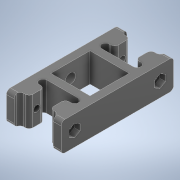
# Autodesk Inventor part: pullitens
Saved by Autodesk Inventor 2022 (Build 260153000, 153)
## iProperties
Created: 2022-03-11
Part Number: pullitens
Material: Genérico
Document SubType Name: Modeling
Designer: JK
Density: 1 g/cm^3
Appearance: Suave - Negro
Author: JK
Autodesk Inventor part; units mm, degrees
ref_plane "YZ Plane" through (0, 0, 0) normal (1, 0, 0) x (0, 1, 0)
ref_plane "XZ Plane" through (0, 0, 0) normal (0, 1, 0) x (-1, 0, 0)
ref_plane "XY Plane" through (0, 0, 0) normal (0, 0, 1) x (1, 0, 0)
sketch "Boceto1" plane through (0, 0, 0) normal (0, 1, 0) x (-1, 0, 0)
  line L0 (-10.15, 10.15) -> (10.15, 10.15)
  line L1 (10.15, 10.15) -> (10.15, -10.15)
  line L2 (10.15, -10.15) -> (-10.15, -10.15)
  line L3 (-10.15, -10.15) -> (-10.15, 10.15)
  line L4 (-10.15, 10.15) -> (10.15, -10.15) construction
  line L5 (10.15, 10.15) -> (-10.15, -10.15) construction
  line L6 (-14.15, 14.15) -> (14.15, 14.15)
  line L7 (14.15, 14.15) -> (14.15, -14.15)
  line L8 (14.15, -14.15) -> (-14.15, -14.15)
  line L9 (-14.15, -14.15) -> (-14.15, 14.15)
  line L10 (-14.15, 14.15) -> (14.15, -14.15) construction
  line L11 (14.15, 14.15) -> (-14.15, -14.15) construction
  point P0 (0, 0)
  dimension "d0" = 20.3
  dimension "d1" = 4
  constraints: 24 end point, 4 midpoint, 4 parallel, 3 perpendicular, 2 horizontal, 1 point on line
  measures "d0" distance of L0.start L0.end
  measures "d1" distance between parallel lines of L0 L6
extrude "Extrusión1" add sketch "Boceto1" along normal blind 15
sketch "Boceto3" plane through (0, 15, 0) normal (0, 1, 0) x (1, 0, 0)
  line L0 (-14.15, -29.15) -> (-10.15, -29.15)
  line L1 (-10.15, -29.15) -> (-10.15, 29.15)
  line L2 (-10.15, 29.15) -> (-14.15, 29.15)
  line L3 (-14.15, 29.15) -> (-14.15, -29.15)
  line L4 (14.15, 29.15) -> (10.15, 29.15)
  line L5 (10.15, 29.15) -> (10.15, -29.15)
  line L6 (10.15, -29.15) -> (14.15, -29.15)
  line L7 (14.15, -29.15) -> (14.15, 29.15)
  line L8 (14.15, 14.15) -> (-14.15, 14.15) projected
  line L9 (-14.15, 14.15) -> (-14.15, -14.15) projected
  line L10 (-14.15, -14.15) -> (14.15, -14.15) projected
  line L11 (14.15, -14.15) -> (14.15, 14.15) projected
  line L12 (10.15, -10.15) -> (-10.15, -10.15) projected
  line L13 (-10.15, -10.15) -> (-10.15, 10.15) projected
  line L14 (-10.15, 10.15) -> (10.15, 10.15) projected
  line L15 (10.15, 10.15) -> (10.15, -10.15) projected
  line L16 (10.15, 10.15) -> (10.15, -10.15) projected
  point P0 (-10.15, 14.15)
  point P1 (-10.15, -14.15)
  point P2 (10.15, 14.15)
  point P3 (10.15, -14.15)
  dimension "d11" = 15
  dimension "d12" = 15
  constraints: 16 end point, 5 collinear, 4 parallel, 2 horizontal, 2 perpendicular, 1 point on line
  measures "d11" distance between parallel lines of L10 L0
  measures "d12" distance between parallel lines of L2 L8
extrude "Extrusión2" add sketch "Boceto3" against normal up to surface (15 mm away) contours L3 L10 L1 L0 | L3 L2 L1 L8 | L10 L7 L6 L5 | L5 L4 L7 L8
sketch "Boceto4" plane through (-14.15, 15, -29.15) normal (-1, 0, 0) x (0, 0, 1)
  circle A0 centre (51.3, -7.5) radius 1.65
  circle A1 centre (7, -7.5) radius 1.65
  line L0 (15, -15) -> (15, 0) projected
  line L1 (0, 0) -> (58.3, 0) projected
  point P0 (29.15, -15)
  point P1 (43.3, 0)
  dimension "d15" = 3.3
  dimension "d16" = 3.3
  dimension "d23" = 8
  dimension "d24" = 8
  dimension "d25" = 7.5
  constraints: 2 centre point, 1 horizontal alignment
  measures "d15" diameter of A1
  measures "d16" diameter of A0
  measures "d23" horizontal distance of A0.centre point (43.3, 0)
  measures "d24" horizontal distance of L0.end A1.centre
  measures "d25" distance from line of A0.centre L1
extrude "Extrusión3" cut sketch "Boceto4" against normal through all
sketch "Boceto5" plane through (-14.15, 15, -29.15) normal (-1, 0, 0) x (0, 0, 1)
  circle A0 centre (51.3, -7.5) radius 1.65 projected
  circle A1 centre (51.3, -7.5) radius 6.5
  point P0 (29.15, -15)
  dimension "d22" = 13
  constraints: 1 centre point, 1 coincident
  measures "d22" diameter of A1
sketch "Boceto6" plane through (-14.15, 15, -29.15) normal (-1, 0, 0) x (0, 0, 1)
  circle A0 centre (29.15, -7.5) radius 2.7
  line L0 (58.3, -15) -> (0, -15) projected
  point P0 (29.15, -15)
  point P1 (29.15, -15)
  dimension "d26" = 5.4
  dimension "d27" = 7.5
  constraints: 1 centre point, 1 midpoint, 1 vertical alignment
  measures "d26" diameter of A0
  measures "d27" distance from line of L0 A0.centre
extrude "Extrusión4" cut sketch "Boceto6" against normal blind 16.8
fillet "Empalme1" radius 2 8 edges at (-12.15, 15, 29.15) (12.15, 15, 29.15) (12.15, 15, -29.15) (-12.15, 15, -29.15) (12.15, 0, 29.15) (-12.15, 0, 29.15) (12.15, 0, -29.15) (-12.15, 0, -29.15)
sketch "Boceto7" plane through (14.15, 15, 27.15) normal (1, 0, 0) x (0, 0, -1)
  circle A0 centre (5, -7.5) radius 1.65 projected
  circle A1 centre (5, -7.5) radius 2.85
  circle A2 centre (49.3, -7.5) radius 1.65 projected
  circle A3 centre (49.3, -7.5) radius 2.85
  line L0 (5, -4.2091) -> (7.85, -5.8546)
  line L1 (7.85, -5.8546) -> (7.85, -9.1454)
  line L2 (7.85, -9.1454) -> (5, -10.7909)
  line L3 (5, -10.7909) -> (2.15, -9.1454)
  line L4 (2.15, -9.1454) -> (2.15, -5.8546)
  line L5 (2.15, -5.8546) -> (5, -4.2091)
  line L6 (49.3, -4.2091) -> (52.15, -5.8546)
  line L7 (52.15, -5.8546) -> (52.15, -9.1454)
  line L8 (52.15, -9.1454) -> (49.3, -10.7909)
  line L9 (49.3, -10.7909) -> (46.45, -9.1454)
  line L10 (46.45, -9.1454) -> (46.45, -5.8546)
  line L11 (46.45, -5.8546) -> (49.3, -4.2091)
  point P0 (27.15, -15)
  dimension "d31" = 5.7
  constraints: 24 end point, 4 coincident, 2 centre point, 2 tangent, 2 vertical, 1 equal radius, 26 other
  measures "d31" diameter of A1
extrude "Extrusión5" cut sketch "Boceto7" against normal blind 3 contours A0 | A1 | L1 L2 A1 | A1 L0 L1 | A1 L5 L0 | L2 L3 A1 | A1 L4 L5 | L3 L4 A1 | A2 | A3 | L7 L8 A3 | A3 L6 L7 | A3 L11 L6 | L8 L9 A3 | A3 L10 L11 | L9 L10 A3
sketch "Boceto9" plane through (0, 0, 0) normal (0, -1, 0) x (1, 0, 0)
  line L0 (-14.15, 27.15) -> (-14.15, -27.15) projected
  line L1 (-10.15, 26.15) -> (-14.15, 26.15)
  line L2 (-14.15, 26.15) -> (-14.15, 18.15)
  line L3 (-14.15, 18.15) -> (-10.15, 18.15)
  line L4 (-10.15, 18.15) -> (-10.15, 26.15)
  line L5 (-10.15, 26.15) -> (-14.15, 18.15) construction
  line L6 (-14.15, 26.15) -> (-10.15, 18.15) construction
  line L7 (-10.15, 14.15) -> (-10.15, 27.15) projected
  line L8 (-10.15, -18.15) -> (-14.15, -18.15)
  line L9 (-14.15, -18.15) -> (-14.15, -26.15)
  line L10 (-14.15, -26.15) -> (-10.15, -26.15)
  line L11 (-10.15, -26.15) -> (-10.15, -18.15)
  line L12 (-10.15, -18.15) -> (-14.15, -26.15) construction
  line L13 (-14.15, -18.15) -> (-10.15, -26.15) construction
  line L14 (-10.15, -27.15) -> (-10.15, -14.15) projected
  line L15 (14.15, 27.15) -> (14.15, -27.15) projected
  line L16 (-14.15, 26.15) -> (14.15, 26.15)
  line L17 (14.15, 26.15) -> (14.15, 18.15)
  line L18 (14.15, 18.15) -> (-14.15, 18.15)
  line L19 (-14.15, 18.15) -> (-14.15, 26.15)
  line L20 (-14.15, -18.15) -> (14.15, -18.15)
  line L21 (14.15, -18.15) -> (14.15, -26.15)
  line L22 (14.15, -26.15) -> (-14.15, -26.15)
  line L23 (-14.15, -26.15) -> (-14.15, -18.15)
  line L24 (-5.4, 26.15) -> (5.4, 26.15)
  line L25 (5.4, 26.15) -> (5.4, 18.15)
  line L26 (5.4, 18.15) -> (-5.4, 18.15)
  line L27 (-5.4, 18.15) -> (-5.4, 26.15)
  line L28 (-5.4, 26.15) -> (5.4, 18.15) construction
  line L29 (5.4, 26.15) -> (-5.4, 18.15) construction
  line L30 (-5.4, -18.15) -> (5.4, -18.15)
  line L31 (5.4, -18.15) -> (5.4, -26.15)
  line L32 (5.4, -26.15) -> (-5.4, -26.15)
  line L33 (-5.4, -26.15) -> (-5.4, -18.15)
  line L34 (-5.4, -18.15) -> (5.4, -26.15) construction
  line L35 (5.4, -18.15) -> (-5.4, -26.15) construction
  line L36 (-10.15, -27.15) -> (-14.15, -27.15) projected
  line L37 (-10.15, -27.15) -> (-10.15, -14.15) projected
  line L38 (10.15, -14.15) -> (-10.15, -14.15) projected
  line L39 (10.15, -14.15) -> (10.15, -27.15) projected
  line L40 (14.15, -27.15) -> (10.15, -27.15) projected
  line L41 (14.15, -27.15) -> (14.15, 27.15) projected
  line L42 (10.15, 27.15) -> (14.15, 27.15) projected
  line L43 (10.15, 27.15) -> (10.15, 14.15) projected
  line L44 (-10.15, 14.15) -> (10.15, 14.15) projected
  line L45 (-10.15, 14.15) -> (-10.15, 27.15) projected
  line L46 (-14.15, 27.15) -> (-10.15, 27.15) projected
  line L47 (-14.15, 27.15) -> (-14.15, -27.15) projected
  line L48 (10.15, 10.15) -> (-10.15, 10.15) projected
  line L49 (10.15, -10.15) -> (10.15, 10.15) projected
  line L50 (-10.15, -10.15) -> (10.15, -10.15) projected
  line L51 (-10.15, 10.15) -> (-10.15, -10.15) projected
  point P0 (0, 0)
  point P1 (-12.15, 22.15)
  point P2 (-12.15, -22.15)
  point P3 (0, 22.15)
  point P4 (0, -22.15)
  point P5 (0, -22.15)
  point P6 (0, 22.15)
  point P7 (10.15, -26.15)
  point P8 (10.15, -18.15)
  point P9 (-5.4, 18.15)
  point P10 (10.15, 18.15)
  point P11 (10.15, 26.15)
  dimension "d37" = 22.15
  dimension "d38" = 8
  dimension "d39" = 22.15
  dimension "d40" = 8
  dimension "d41" = 10.8
  dimension "d42" = 8
  constraints: 64 end point, 12 parallel, 10 midpoint, 7 collinear, 6 horizontal, 6 perpendicular, 5 point on line, 2 vertical alignment
  measures "d37" vertical distance of point (0, 0) point (-12.15, 22.15)
  measures "d38" distance between parallel lines of L3 L1
  measures "d39" vertical distance of point (0, 0) point (-12.15, -22.15)
  measures "d40" distance between parallel lines of L10 L8
  measures "d41" distance between parallel lines of L27 L25
  measures "d42" distance of L30.end L31.end
extrude "Extrusión7" add sketch "Boceto9" against normal up to surface (15 mm away) contours L16 L27 L18 L4 | L20 L33 L22 L11 | L16 L43 L18 L25 | L20 L39 L22 L31
sketch "Boceto10" plane through (14.15, 15, 27.15) normal (1, 0, 0) x (0, 0, -1)
  circle A0 centre (5, -7.5) radius 1.65 projected
  circle A1 centre (49.3, -7.5) radius 1.65 projected
  point P0 (27.15, -15)
extrude "Extrusión8" cut sketch "Boceto10" against normal through all
fillet "Empalme2" radius 2 20 edges at (10.15, 7.5, 18.15) (10.15, 7.5, 26.15) (10.15, 7.5, -18.15) (10.15, 7.5, -26.15) (10.15, 7.5, -14.15) (-10.15, 7.5, -14.15) (-10.15, 7.5, -18.15) (-10.15, 7.5, -26.15) (-10.15, 7.5, 18.15) (-10.15, 7.5, 26.15) (-10.15, 7.5, 14.15) (10.15, 7.5, 14.15) (5.4, 7.5, 18.15) (5.4, 7.5, 26.15) (-5.4, 7.5, 26.15) (-5.4, 7.5, 18.15) (-5.4, 7.5, -18.15) (-5.4, 7.5, -26.15) (5.4, 7.5, -18.15) (5.4, 7.5, -26.15)
sketch "Boceto8" plane through (-14.15, 15, -27.15) normal (-1, 0, 0) x (0, 0, 1)
  circle A0 centre (49.3, -7.5) radius 1.65 projected
  circle A1 centre (49.3, -7.5) radius 3.05
  circle A2 centre (5, -7.5) radius 1.65 projected
  circle A3 centre (5, -7.5) radius 3.05
  point P0 (27.15, -15)
  dimension "d34" = 6.1
  constraints: 2 centre point, 2 coincident, 1 equal radius
  measures "d34" diameter of A1
